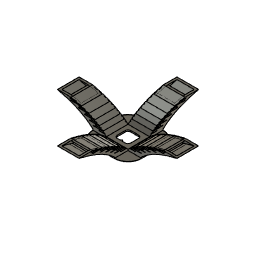
bear_overhang_small_50-75 (Autodesk Fusion 360 design; units mm, degrees)
Autodesk Fusion 360 part; units mm, degrees
sketch "arm" plane through (0, 0, 0) normal (0, 1, 0) x (1, 0, 0) in component "bear_overhang_small_50-75"
  line L0 (18, 0) -> (8, 0)
  line L1 (23.4782, -4.2) -> (26.9423, -6.2)
  line L2 (18, 0) -> (20.6219, -2.2)
  line L3 (20.6219, -2.2) -> (23.4782, -4.2)
  line L4 (0, 1) -> (0, 0)
  line L5 (0, 0) -> (0, -27.1786) construction
  line L6 (16.9423, -6.2) -> (13.4782, -4.2)
  line L7 (26.9423, -6.2) -> (16.9423, -6.2) construction
  line L8 (23.4782, -4.2) -> (13.4782, -4.2) construction
  line L9 (20.6219, -2.2) -> (10.6219, -2.2) construction
  line L10 (13.4782, -4.2) -> (10.6219, -2.2)
  line L11 (10.6219, -2.2) -> (8, 0)
  line L12 (26.9423, -6.2) -> (31.2313, -8.2)
  line L13 (31.2313, -8.2) -> (36.7262, -10.2)
  line L14 (16.9423, -6.2) -> (21.2313, -8.2)
  line L15 (21.2313, -8.2) -> (26.7262, -10.2)
  line L16 (31.2313, -8.2) -> (21.2313, -8.2) construction
  line L17 (8, 0) -> (0, 0)
  line L18 (0, 1) -> (18, 1)
  line L19 (36.7262, -10.2) -> (44.1903, -12.2)
  line L20 (44.1903, -12.2) -> (34.1903, -12.2)
  line L21 (26.7262, -10.2) -> (36.7262, -10.2) construction
  line L22 (26.7262, -10.2) -> (34.1903, -12.2)
  line L23 (16.3287, 0) -> (18.9506, -2.2)
  line L24 (18.9506, -2.2) -> (21.8069, -4.2)
  line L25 (21.8069, -4.2) -> (25.271, -6.2)
  line L26 (25.271, -6.2) -> (29.56, -8.2)
  line L27 (29.56, -8.2) -> (35.0549, -10.2)
  line L28 (35.0549, -10.2) -> (42.519, -12.2)
  line L29 (9.6713, 0) -> (12.2932, -2.2)
  line L30 (12.2932, -2.2) -> (15.1495, -4.2)
  line L31 (15.1495, -4.2) -> (18.6136, -6.2)
  line L32 (18.6136, -6.2) -> (22.9026, -8.2)
  line L33 (22.9026, -8.2) -> (28.3975, -10.2)
  line L34 (28.3975, -10.2) -> (35.8616, -12.2)
  line L35 (18, 1) -> (18, 0)
  dimension "d9" = 2.2
  dimension "d10" = 2
  dimension "d13" = 2
  dimension "d24" = 50
  dimension "d25" = 55
  dimension "d26" = 60
  dimension "d45" = 7.6
  dimension "d46" = 7.6019
  dimension "d50" = 65
  dimension "d51" = 70
  dimension "d52" = 2
  dimension "d53" = 2
  dimension "d54" = 6.6254
  dimension "d55" = 7.0171
  dimension "d78" = 10
  dimension "d79" = 8
  dimension "d85" = 5.9118
  dimension "d99" = 75
  dimension "d100" = 10.1153
  dimension "d101" = 2
  dimension "d124" = 1.6713
  dimension "d125" = 1.6713
  dimension "d129" = 1
  constraint horizontal L7
  constraint horizontal L8
  constraint horizontal L9
  constraint horizontal L0
  constraint coincident L4.end L5.start
  constraint horizontal L16
  constraint perpendicular L5 L17
  constraint parallel L0 L17
  constraint equal L0 L9
  constraint perpendicular L4 L17
  constraint perpendicular L5 L18
  constraint horizontal L21
  constraint horizontal L20
  constraint equal L8 L9
  constraint equal L7 L8
  constraint equal L7 L16
  constraint equal L16 L21
  constraint equal L20 L21
  constraint coincident L0 L23.start
  constraint coincident L9 L23.end
  constraint coincident L8 L24.end
  constraint coincident L7 L25.end
  constraint parallel L2 L23
  constraint parallel L3 L24
  constraint parallel L1 L25
  constraint coincident L16 L26.end
  constraint coincident L21 L27.end
  constraint coincident L20 L28.end
  constraint parallel L12 L26
  constraint parallel L13 L27
  constraint parallel L19 L28
  constraint coincident L0 L29.start
  constraint coincident L9 L29.end
  constraint coincident L8 L30.end
  constraint coincident L7 L31.end
  constraint coincident L16 L32.end
  constraint coincident L21 L33.end
  constraint coincident L20 L34.end
  constraint parallel L11 L29
  constraint parallel L10 L30
  constraint parallel L6 L31
  constraint parallel L14 L32
  constraint parallel L15 L33
  constraint parallel L22 L34
  constraint perpendicular L18 L35
  measures "d9" vertical distance of L2.end L0.start
  measures "d10" vertical distance of L2.end L1.start
  measures "d13" vertical distance of L1.end L1.start
  measures "d24" angle of L2 L5
  measures "d25" angle of L3 L5
  measures "d26" angle of L1 L5
  measures "d50" angle of L5 L12
  measures "d51" angle of L5 L13
  measures "d52" vertical distance of L1.end L12.end
  measures "d53" vertical distance of L13.end L12.end
  measures "d78" distance of L0.start L0.end
  measures "d79" distance of L4.end L0.end
  measures "d99" angle of L5 L19
  measures "d101" vertical distance of L13.end L19.end
  measures "d124" distance of L0.start L23.start
  measures "d125" distance of L0.end L29.start
  measures "d129" distance of L4.end L4.start
extrude "Extrude1" add sketch "arm" along normal mid plane 16 makes body 1 in component "bear_overhang_small_50-75"
extrude "Extrude5" cut sketch "arm" along normal up to surface (12.6574 mm away) from surface at -6.3287 contours L0 L20 L23 L24 L25 L26 L27 L28 L29 L30 L31 L32 L33 L34 bodies 1 in component "bear_overhang_small_50-75"
sketch "angle_indication" plane through (0, -8, 0) normal (0, -1, 0) x (1, 0, 0) in component "bear_overhang_small_50-75"
  line L0 (17.6219, 2.2) -> (10.6219, 2.2)
  line L1 (20.4782, 4.2) -> (13.4782, 4.2)
  line L2 (23.9423, 6.2) -> (16.9423, 6.2)
  line L3 (28.2313, 8.2) -> (21.2313, 8.2)
  line L4 (17.6219, 2.2) -> (17.9075, 2.4)
  line L5 (17.9075, 2.4) -> (10.9075, 2.4)
  line L6 (20.4782, 4.2) -> (20.8246, 4.4)
  line L7 (20.8246, 4.4) -> (13.8246, 4.4)
  line L8 (23.9423, 6.2) -> (24.3712, 6.4)
  line L9 (24.3712, 6.4) -> (17.3712, 6.4)
  line L10 (28.2313, 8.2) -> (28.7808, 8.4)
  line L11 (28.7808, 8.4) -> (21.7808, 8.4)
  line L12 (13.4782, 4.2) -> (10.6219, 2.2)
  line L13 (16.9423, 6.2) -> (13.4782, 4.2)
  line L14 (21.2313, 8.2) -> (16.9423, 6.2)
  line L15 (26.7262, 10.2) -> (21.2313, 8.2)
  line L16 (34.1903, 12.2) -> (26.7262, 10.2)
  line L17 (33.7262, 10.2) -> (26.7262, 10.2)
  line L18 (27.4726, 10.4) -> (34.4726, 10.4)
  line L19 (34.4726, 10.4) -> (33.7262, 10.2)
  line L20 (12.05, 3.2) -> (16.05, 3.2)
  line L21 (16.05, 3.2) -> (16.3356, 3.4)
  line L22 (16.3356, 3.4) -> (12.3356, 3.4)
  line L23 (15.2102, 5.2) -> (19.2102, 5.2)
  line L24 (19.2102, 5.2) -> (19.5566, 5.4)
  line L25 (19.5566, 5.4) -> (15.5566, 5.4)
  line L26 (19.0868, 7.2) -> (23.0868, 7.2)
  line L27 (23.0868, 7.2) -> (23.5157, 7.4)
  line L28 (23.5157, 7.4) -> (19.5157, 7.4)
  line L29 (23.9787, 9.2) -> (27.9787, 9.2)
  line L30 (27.9787, 9.2) -> (28.5282, 9.4)
  line L31 (28.5282, 9.4) -> (24.5282, 9.4)
  line L32 (30.4583, 11.2) -> (34.4583, 11.2)
  line L33 (34.4583, 11.2) -> (35.2047, 11.4)
  line L34 (35.2047, 11.4) -> (31.2047, 11.4)
  line L35 (10.6219, 2.2) -> (8, 0)
  line L36 (9.3109, 1.1) -> (13.3109, 1.1)
  line L37 (13.3109, 1.1) -> (13.5493, 1.3)
  line L38 (13.5493, 1.3) -> (9.5493, 1.3)
  point P0 (20.6219, 2.2)
  point P1 (23.4782, 4.2)
  point P2 (26.9423, 6.2)
  point P3 (31.2313, 8.2)
  point P4 (36.7262, 10.2)
  dimension "d68" = 0.2
  dimension "d69" = 0.2
  dimension "d70" = 0.2
  dimension "d71" = 0.2
  dimension "d102" = 0.2
  dimension "d116" = 0.2
  dimension "d117" = 0.2
  dimension "d118" = 0.2
  dimension "d119" = 0.2
  dimension "d122" = 0.2
  dimension "d132" = 7
  dimension "d141" = 0.2
  dimension "d142" = 4
  constraint parallel L0 L5
  constraint parallel L1 L7
  constraint parallel L2 L9
  constraint parallel L3 L11
  constraint coincident L11.end L15
  constraint coincident L3.end L14.start
  constraint coincident L2.end L13.start
  constraint coincident L1.end L12.start
  constraint coincident L0.end L12.end
  constraint parallel L4 L12
  constraint parallel L6 L13
  constraint coincident L9.end L14
  constraint coincident L7.end L13
  constraint coincident L5.end L12
  constraint coincident L15.start L16.end
  constraint coincident L16 L18.start
  constraint parallel L17 L18
  constraint parallel L16 L19
  constraint midpoint L12 L20.start
  constraint horizontal L20
  constraint parallel L12 L21
  constraint parallel L20 L22
  constraint coincident L12 L22.end
  constraint midpoint L13 L23.start
  constraint parallel L13 L24
  constraint coincident L13 L25.end
  constraint parallel L23 L25
  constraint midpoint L14 L26.start
  constraint coincident L14 L28.end
  constraint midpoint L15 L29.start
  constraint coincident L15 L31.end
  constraint midpoint L16 L32.start
  constraint parallel L32 L34
  constraint coincident L16 L34.end
  constraint parallel L16 L33
  constraint parallel L26 L28
  constraint parallel L8 L14
  constraint parallel L14 L27
  constraint parallel L15 L30
  constraint horizontal L0
  constraint horizontal L1
  constraint horizontal L2
  constraint horizontal L3
  constraint horizontal L17
  constraint parallel L10 L15
  constraint horizontal L23
  constraint horizontal L26
  constraint horizontal L29
  constraint horizontal L32
  constraint equal L29 L32
  constraint equal L26 L29
  constraint equal L23 L26
  constraint equal L20 L23
  constraint equal L0 L1
  constraint equal L1 L2
  constraint equal L2 L3
  constraint equal L3 L17
  constraint midpoint L35 L36.start
  constraint horizontal L36
  constraint parallel L35 L37
  constraint coincident L35 L38.end
  constraint parallel L36 L38
  constraint equal L20 L36
  measures "d68" distance of L0 L5
  measures "d69" distance of L1 L7
  measures "d70" distance of L2 L9
  measures "d71" distance of L3 L11
  measures "d102" distance of L17 L18
  measures "d116" distance of L20 L22
  measures "d117" distance of L23 L25
  measures "d118" distance of L26 L28
  measures "d119" distance of L29 L31
  measures "d122" distance of L32 L34
  measures "d132" distance of L0.start L0.end
  measures "d141" distance of L36 L38
  measures "d142" distance of L36.start L36.end
extrude "Extrude2" cut sketch "angle_indication" against normal blind 0.4071 bodies 1 in component "bear_overhang_small_50-75"
mirror "Mirror1" about plane through (0, 0, 0) normal (0, 1, 0) of "Extrude2" in component "bear_overhang_small_50-75"
pattern_circular "C-Pattern1" count 4 over 360 about axis through (0, 0, 1.75) along (0, 0, 1) of bodies 1 makes body 2 at (8, 16.3904, 1.1667) makes body 3 at (-16.3904, -8, 1.1667) makes body 4 at (2.6667, -6, -1) in component "bear_overhang_small_50-75"
combine "Combine1" operation add target body 1 tool bodies 4 3 2 in component "bear_overhang_small_50-75"
sketch "orientation_mark" plane through (0, 0, -1) normal (0, 0, -1) x (1, 0, 0) in component "bear_overhang_small_50-75"
  arc A0 (8, -18) -> (18, -8) centre (8, -8) ccw
  arc A1 (18, 8) -> (8, 18) centre (8, 8) ccw
  arc A2 (-8, 18) -> (-18, 8) centre (-8, 8) ccw
  arc A3 (-18, -8) -> (-8, -18) centre (-8, -8) ccw
  line L0 (0, 18) -> (0, -18) construction
  line L1 (-18, 0) -> (18, 0) construction
  line L2 (3, -5) -> (-3, -5)
  line L3 (-5, -3) -> (-5, 3)
  line L4 (-3, 5) -> (3, 5)
  line L5 (5, 3) -> (5, -3)
  arc A4 (3, -5) -> (5, -3) centre (3, -3) ccw
  arc A5 (5, 3) -> (3, 5) centre (3, 3) ccw
  arc A6 (-3, 5) -> (-5, 3) centre (-3, 3) ccw
  arc A7 (-5, -3) -> (-3, -5) centre (-3, -3) ccw
  line L6 (-0.7002, 5) -> (0, 4)
  line L7 (0, 4) -> (0.7002, 5)
  line L8 (8, -8) -> (18, -8)
  line L9 (18, -8) -> (18, 8)
  line L10 (18, 8) -> (8, 8)
  line L11 (8, 8) -> (8, 18)
  line L12 (8, 18) -> (-8, 18)
  line L13 (-8, 18) -> (-8, 8)
  line L14 (-8, 8) -> (-18, 8)
  line L15 (-18, 8) -> (-18, -8)
  line L16 (-18, -8) -> (-8, -8)
  line L17 (-8, -8) -> (-8, -18)
  line L18 (-8, -18) -> (8, -18)
  line L19 (8, -18) -> (8, -8)
  point P0 (-8, 18)
  dimension "d134" = 2
  dimension "d137" = 70
  dimension "d138" = 1
  dimension "d139" = 3
  constraint horizontal L2
  constraint vertical L3
  constraint horizontal L4
  constraint vertical L5
  constraint tangent L2 A4
  constraint tangent L5 A4
  constraint tangent L5 A5
  constraint tangent L4 A5
  constraint equal A4 A5
  constraint tangent L4 A6
  constraint tangent L3 A6
  constraint equal A4 A6
  constraint tangent L2 A7
  constraint tangent L3 A7
  constraint equal A4 A7
  constraint equal L2 L5
  constraint symmetric L1 L2 L4
  constraint coincident L4 L6.start
  constraint coincident L0 L6.end
  constraint coincident L4 L7.end
  constraint symmetric L0 L6 L7
  constraint coincident A3.start L15.end
  constraint coincident A3.end L17.end
  constraint coincident A2 L14.end
  constraint coincident A2 P0
  constraint midpoint L0.start L12
  constraint midpoint L0.end L18
  constraint midpoint L1.start L15
  constraint midpoint L1.end L9
  constraint coincident A1.end L11.end
  constraint coincident A1.start L9.end
  constraint coincident A0.start L18.end
  constraint coincident A0.end L8.end
  constraint tangent A1 L12
  constraint tangent A2 L12
  constraint tangent A3 L15
  constraint tangent A0 L18
  measures "d134" radius of A4
  measures "d137" angle of L6 L7
  measures "d138" distance of L4 L6.end
  measures "d139" distance of L3 L13
extrude "Extrude3" add sketch "orientation_mark" against normal blind 0.2 contours A0 L8 L19 | A3 L16 L17 | A1 L10 L11 | A2 L13 L14 bodies 1 in component "bear_overhang_small_50-75"
extrude "Extrude4" cut sketch "orientation_mark" against normal blind 3 contours L2 L3 L4 L5 A4 A5 A6 A7 L6 L7 bodies 1 in component "bear_overhang_small_50-75"
component "bear_overhang_small_50-75" placed x (1, 0, 0) y (0, 1, 0) z (0, 0, 1) at (0, 0, 0)
equation "d9 = layer_height * 11"
equation "d10 = layer_height * 10"
equation "d13 = layer_height * 10"
equation "d31 = arm_width"
equation "layer_height = 0.2 mm"
equation "arm_width = 16 mm"
equation "arm_support_width = arm_width / 3"
equation "d52 = layer_height * 10"
equation "d53 = layer_height * 10"
equation "arm_layer_length = e_width + ( num_perimeters * 2 - 1 ) * e_spacing"
equation "d68 = layer_height"
equation "d69 = layer_height"
equation "d70 = layer_height"
equation "d71 = layer_height"
equation "d72 = -e_spacing"
equation "d75 = -layer_height"
equation "d79 = arm_width / 2"
equation "e_width = 0.45 mm"
equation "e_spacing = 0.4071 mm"
equation "num_perimeters = 4"
equation "d101 = layer_height * 10"
equation "d102 = layer_height"
equation "d116 = layer_height"
equation "d117 = layer_height"
equation "d118 = layer_height"
equation "d119 = layer_height"
equation "d122 = layer_height"
equation "d124 = e_width + ( num_perimeters - 1 ) * e_spacing"
equation "d125 = e_width + ( num_perimeters - 1 ) * e_spacing"
equation "d126 = -e_width - ( num_perimeters - 1 ) * e_spacing"
equation "d127 = -e_width - ( num_perimeters - 1 ) * e_spacing"
equation "d141 = layer_height"
